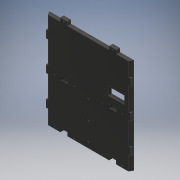
# Autodesk Inventor part: BA04
Saved by Autodesk Inventor 2017 (Build 210142000, 142)
## iProperties
Created: 2019-05-22
Part Number: BA04
Material: Wood (Cherry)
Document SubType Name: Modeling
Designer: Dell
Density: 0.63 g/cm^3
Appearance: Smooth - Black
Mass: 809.541 g
Surface Area: 2261.79 cm^2
Volume: 1284.98 cm^3
Author: Dell
Autodesk Inventor part; units mm, degrees
ref_plane "YZ Plane" through (0, 0, 0) normal (1, 0, 0) x (0, 1, 0)
ref_plane "XZ Plane" through (0, 0, 0) normal (0, 1, 0) x (-1, 0, 0)
ref_plane "XY Plane" through (0, 0, 0) normal (0, 0, 1) x (1, 0, 0)
sketch "Sketch1" plane through (0, 0, 0) normal (0, 0, 1) x (1, 0, 0)
  line L0 (0, 0) -> (303.5592, 0)
  line L1 (303.5592, 0) -> (455.3388, -262.89) construction
  line L2 (455.3388, -262.89) -> (404.5388, -350.8782)
  line L3 (404.5388, -350.8782) -> (-50.8, -87.9882) construction
  line L4 (-50.8, -87.9882) -> (0, 0) construction
  line L5 (0, 0) -> (7.3323, -12.7)
  line L6 (7.3323, -12.7) -> (296.2269, -12.7)
  line L7 (296.2269, -12.7) -> (303.5592, 0)
  dimension "d0" = 525.78
  dimension "d1" = 101.6
  dimension "d2" = 120
  dimension "d3" = 12.7
  dimension "d4" = 60
  dimension "d5" = 60
  constraints: 16 end point, 2 equal length, 2 horizontal, 2 perpendicular
  measures "d0" distance of L2.end L3.end
  measures "d1" distance of L3.end L0.start
  measures "d2" angle of L0 L4
  measures "d3" distance between parallel lines of L0 L6
  measures "d4" angle of L0 L5
  measures "d5" angle of L0 L7
extrude "Extrusion1" add sketch "Sketch1" along normal blind 342.9
sketch "Sketch2" plane through (7.3323, -12.7, 0) normal (0, -1, 0) x (1, 0, 0)
  line L0 (296.2269, 342.9) -> (-7.3323, 342.9) projected
  line L1 (43.4677, 342.9) -> (68.8677, 342.9)
  line L2 (68.8677, 342.9) -> (68.8677, 355.6)
  line L3 (68.8677, 355.6) -> (43.4677, 355.6)
  line L4 (43.4677, 355.6) -> (43.4677, 342.9)
  line L5 (220.0269, 342.9) -> (245.4269, 342.9)
  line L6 (245.4269, 342.9) -> (245.4269, 355.6)
  line L7 (245.4269, 355.6) -> (220.0269, 355.6)
  line L8 (220.0269, 355.6) -> (220.0269, 342.9)
  line L9 (-7.3323, 0) -> (-7.3323, 342.9) projected
  line L10 (296.2269, 0) -> (296.2269, 342.9) projected
  circle A0 centre (56.1677, 349.25) radius 2.25
  circle A1 centre (232.7269, 349.25) radius 2.25
  point P0 (56.1677, 355.6)
  point P1 (232.7269, 355.6)
  point P2 (68.8677, 349.25)
  point P3 (245.4269, 349.25)
  dimension "d8" = 25.4
  dimension "d9" = 12.7
  dimension "d10" = 25.4
  dimension "d11" = 12.7
  dimension "d12" = 50.8
  dimension "d13" = 50.8
  dimension "d16" = 4.5
  dimension "d17" = 4.5
  constraints: 16 end point, 4 midpoint, 4 parallel, 2 centre point, 2 horizontal, 2 horizontal alignment, 2 perpendicular, 2 point on line, 2 vertical alignment
  measures "d8" distance of L3.end L2.end
  measures "d9" distance of L2.end L1.end
  measures "d10" distance of L7.end L6.end
  measures "d11" distance of L6.end L5.end
  measures "d12" distance between parallel lines of L9 L4
  measures "d13" distance between parallel lines of L10 L6
  measures "d16" diameter of A0
  measures "d17" diameter of A1
extrude "Extrusion2" add sketch "Sketch2" against normal blind 12.7
ref_plane "Work Plane1" through (0, 0, 292.1) normal (0, 0, 1) x (1, 0, 0)
sketch "Sketch3" plane through (0, 0, 292.1) normal (0, 0, 1) x (1, 0, 0)
  line L0 (0, 0) -> (303.5592, 0) projected
  line L1 (0, 0) -> (0, -12.7)
  line L2 (296.2269, -12.7) -> (7.3323, -12.7) projected
  line L3 (0, -12.7) -> (7.3323, -12.7)
  line L4 (7.3323, -12.7) -> (0, 0) projected
  constraints: 4 end point, 1 perpendicular, 1 vertical
extrude "Extrusion3" add sketch "Sketch3" against normal blind 25.4
ref_plane "Work Plane2" through (0, 0, 50.8) normal (0, 0, -1) x (-1, 0, 0)
sketch "Sketch4" plane through (0, 0, 50.8) normal (0, 0, -1) x (-1, 0, 0)
  line L0 (0, -12.7) -> (0, 0) projected
  line L1 (-7.3323, -12.7) -> (0, 0) projected
  line L2 (-7.3323, -12.7) -> (0, -12.7) projected
extrude "Extrusion4" add sketch "Sketch4" against normal blind 25.4
ref_plane "Work Plane3" through (0, 0, 171.45) normal (0, 0, -1) x (-1, 0, 0)
sketch "Sketch5" plane through (0, 0, 171.45) normal (0, 0, -1) x (-1, 0, 0)
  line L0 (0, 0) -> (0, -12.7) projected
  line L1 (0, -12.7) -> (-7.3323, -12.7) projected
  line L2 (0, 0) -> (-7.3323, -12.7) projected
extrude "Extrusion5" add sketch "Sketch5" along normal mid plane 25.4
ref_plane "Work Plane4" through (151.7796, -12.7, 342.9) normal (-1, 0, 0) x (0, 0, 1)
mirror "Mirror1" about plane through (151.7796, -12.7, 342.9) normal (-1, 0, 0) of "Extrusion5", "Extrusion4", "Extrusion3"
sketch "Sketch6" plane through (0, 0, 0) normal (0, 0, -1) x (-1, 0, 0)
  line L0 (-76.9796, -12.7) -> (-76.9796, 0)
  line L1 (-76.9796, -6.35) -> (-64.2796, -6.35) construction
  circle A0 centre (-64.2796, -6.35) radius 2.25
  line L2 (-64.2796, -6.35) -> (-64.2796, 0) construction
  line L3 (-51.5796, -12.7) -> (-76.9796, -12.7)
  line L4 (-76.9796, 0) -> (-51.5796, 0)
  line L5 (-51.5796, 0) -> (-51.5796, -12.7)
  line L6 (-226.5796, 0) -> (-226.5796, -12.7)
  line L7 (-239.2796, 0) -> (-64.2796, 0) construction
  line L8 (-251.9796, 0) -> (-226.5796, 0)
  line L9 (-251.9796, -12.7) -> (-251.9796, 0)
  circle A1 centre (-239.2796, -6.35) radius 2.25
  line L10 (-239.2796, -6.35) -> (-239.2796, 0) construction
  line L11 (-239.2796, -6.35) -> (-226.5796, -6.35) construction
  line L12 (-226.5796, -12.7) -> (-251.9796, -12.7)
  line L13 (0, 0) -> (-303.5592, 0)
  line L14 (0, 0) -> (-303.5592, 0) projected
  point P0 (-151.7796, 0)
  dimension "d26" = 25.4
  dimension "d27" = 12.7
  dimension "d28" = 12.7
  dimension "d29" = 25.4
  dimension "d30" = 175
  dimension "d31" = 4.5
  dimension "d32" = 4.5
  constraints: 28 end point, 7 midpoint, 6 perpendicular, 4 parallel, 4 point on line, 2 centre point
  measures "d26" distance of L0.end L5.start
  measures "d27" distance of L5.start L3.start
  measures "d28" distance of L9.start L8.start
  measures "d29" distance of L8.start L6.start
  measures "d30" distance of L7.start L2.end
  measures "d31" diameter of A1
  measures "d32" diameter of A0
extrude "Extrusion6" cut sketch "Sketch6" against normal blind 12.7 contours L0 L4 L5 L3 | A0 | L6 L12 L9 L8 | A1
sketch "Sketch7" plane through (227.3592, -12.7, 355.6) normal (0, -1, 0) x (1, 0, 0)
  line L0 (-175.7796, -181.45) -> (-150.3796, -181.45)
  line L1 (-150.3796, -181.45) -> (-150.3796, -194.15)
  line L2 (-150.3796, -194.15) -> (-175.7796, -194.15)
  line L3 (-175.7796, -194.15) -> (-175.7796, -181.45)
  line L4 (-0.7796, -181.45) -> (24.6204, -181.45)
  line L5 (24.6204, -181.45) -> (24.6204, -194.15)
  line L6 (24.6204, -194.15) -> (-0.7796, -194.15)
  line L7 (-0.7796, -194.15) -> (-0.7796, -181.45)
  line L8 (-175.7796, -342.9) -> (-150.3796, -342.9) projected
  line L9 (-0.7796, -342.9) -> (24.6204, -342.9) projected
  line L10 (-227.3592, -171.45) -> (-220.0269, -171.45) projected
  point P0 (-227.3592, -355.6)
  point P1 (-163.0796, -194.15)
  point P2 (-163.0796, -342.9)
  point P3 (11.9204, -194.15)
  point P4 (11.9204, -342.9)
  dimension "d36" = 25.4
  dimension "d37" = 12.7
  dimension "d38" = 25.4
  dimension "d39" = 12.7
  dimension "d40" = 10
  constraints: 16 end point, 4 midpoint, 4 parallel, 2 horizontal, 2 perpendicular, 2 vertical alignment, 1 horizontal alignment
  measures "d36" distance of L1.end L2.end
  measures "d37" distance of L0.end L1.end
  measures "d38" distance of L5.end L6.end
  measures "d39" distance of L4.end L5.end
  measures "d40" distance between parallel lines of L10 L0
extrude "Extrusion7" cut sketch "Sketch7" against normal through all
sketch "Sketch8" plane through (227.3592, -12.7, 355.6) normal (0, -1, 0) x (1, 0, 0)
  line L0 (-150.3796, -355.6) -> (-0.7796, -355.6) construction
  line L1 (-100.9796, -355.6) -> (-50.1796, -355.6) construction
  line L2 (-50.1796, -355.6) -> (-50.1796, -181.45) construction
  line L3 (-50.1796, -181.45) -> (-100.9796, -181.45) construction
  line L4 (-100.9796, -181.45) -> (-100.9796, -355.6) construction
  circle A0 centre (-75.5796, -268.525) radius 4
  circle A1 centre (-75.5796, -201.45) radius 4
  circle A2 centre (-75.5796, -335.6) radius 4
  line L5 (-0.7796, -355.6) -> (-150.3796, -355.6)
  line L6 (-0.7796, -355.6) -> (-150.3796, -355.6) projected
  circle A3 centre (-126.3796, -187.8) radius 2.25
  circle A4 centre (-126.3796, -349.25) radius 2.25
  circle A5 centre (-24.7796, -349.25) radius 2.25
  circle A6 centre (-24.7796, -187.8) radius 2.25
  line L7 (-150.3796, -181.45) -> (-150.3796, -194.15) projected
  line L8 (-150.3796, -342.9) -> (-150.3796, -355.6) projected
  point P0 (-75.5796, -355.6)
  point P1 (-75.5796, -355.6)
  point P2 (-75.5796, -355.6)
  point P3 (-100.9796, -268.525)
  point P4 (-150.3796, -187.8)
  point P5 (-150.3796, -349.25)
  dimension "d44" = 8
  dimension "d45" = 8
  dimension "d46" = 8
  dimension "d47" = 20
  dimension "d48" = 20
  dimension "d49" = 50.8
  dimension "d59" = 4.5
  dimension "d60" = 4.5
  dimension "d61" = 4.5
  dimension "d62" = 4.5
  dimension "d63" = 25.4
  dimension "d64" = 25.4
  constraints: 12 end point, 7 centre point, 7 midpoint, 6 horizontal alignment, 5 vertical alignment, 2 coincident, 2 parallel, 1 horizontal, 1 perpendicular, 1 point on line
  measures "d44" diameter of A0
  measures "d45" diameter of A1
  measures "d46" diameter of A2
  measures "d47" distance from line of L3 A1.centre
  measures "d48" distance from line of L0 A2.centre
  measures "d49" distance of L2.end L3.end
  measures "d59" diameter of A3
  measures "d60" diameter of A4
  measures "d61" diameter of A5
  measures "d62" diameter of A6
  measures "d63" distance from line of A3.centre L4
  measures "d64" distance from line of A6.centre L2
extrude "Extrusion8" cut sketch "Sketch8" against normal through all
sketch "Sketch9" plane through (227.3592, -12.7, 355.6) normal (0, -1, 0) x (1, 0, 0)
  circle A0 centre (-197.9032, -187.8) radius 2.25
  circle A1 centre (46.744, -187.8) radius 2.25
  circle A2 centre (-197.9032, -349.25) radius 2.25
  circle A3 centre (46.744, -349.25) radius 2.25
  line L0 (-175.7796, -194.15) -> (-175.7796, -181.45) projected
  line L1 (-175.7796, -355.6) -> (-175.7796, -342.9) projected
  line L2 (24.6204, -342.9) -> (24.6204, -355.6) projected
  line L3 (-175.7796, -355.6) -> (-220.0269, -355.6) projected
  line L4 (68.8677, -355.6) -> (24.6204, -355.6) projected
  line L5 (24.6204, -181.45) -> (24.6204, -194.15) projected
  point P0 (-227.3592, -355.6)
  point P1 (-175.7796, -187.8)
  point P2 (-175.7796, -349.25)
  point P3 (24.6204, -349.25)
  point P4 (-197.9032, -355.6)
  point P5 (46.744, -355.6)
  point P6 (24.6204, -187.8)
  dimension "d52" = 4.5
  dimension "d54" = 4.5
  dimension "d55" = 4.5
  dimension "d56" = 4.5
  constraints: 6 midpoint, 4 centre point, 4 horizontal alignment, 4 vertical alignment
  measures "d52" diameter of A0
  measures "d54" diameter of A1
  measures "d55" diameter of A2
  measures "d56" diameter of A3
extrude "Extrusion9" cut sketch "Sketch9" against normal through all
sketch "Sketch11" plane through (227.3592, -12.7, 355.6) normal (0, -1, 0) x (1, 0, 0)
  line L0 (-85.5796, -112.7) -> (-65.5796, -112.7)
  line L1 (-65.5796, -112.7) -> (-65.5796, -122.7)
  line L2 (-65.5796, -122.7) -> (-85.5796, -122.7)
  line L3 (-85.5796, -122.7) -> (-85.5796, -112.7)
  line L4 (-151.1592, -12.7) -> (0, -12.7) projected
  point P0 (-227.3592, -355.6)
  point P1 (-75.5796, -112.7)
  point P2 (-75.5796, -12.7)
  dimension "d65" = 20
  dimension "d66" = 10
  dimension "d67" = 100
  constraints: 8 end point, 2 midpoint, 2 parallel, 1 horizontal, 1 perpendicular, 1 vertical alignment
  measures "d65" distance of L1.end L2.end
  measures "d66" distance of L0.end L1.end
  measures "d67" distance between parallel lines of L4 L0
extrude "Extrusion10" [suppressed]
sketch "Sketch12" plane through (76.2, 0, 342.9) normal (0, 1, 0) x (1, 0, 0)
  line L0 (206.2304, 143.75) -> (176.2304, 143.75)
  line L1 (176.2304, 143.75) -> (176.2304, 128.75)
  line L2 (176.2304, 128.75) -> (206.2304, 128.75)
  line L3 (206.2304, 128.75) -> (206.2304, 143.75)
  line L4 (0.7796, 168.75) -> (-24.6204, 168.75) projected
  line L5 (220.0269, 50.8) -> (220.0269, 0) projected
  point P0 (-76.2, 342.9)
  dimension "d70" = 30
  dimension "d71" = 15
  dimension "d72" = 25
  dimension "d76" = 13.7965
  constraints: 8 end point, 2 parallel, 1 horizontal, 1 perpendicular
  measures "d70" distance of L2.end L1.end
  measures "d71" distance of L1.end L0.end
  measures "d72" distance between parallel lines of L4 L0
  measures "d76" distance between parallel lines of L5 L3
extrude "Extrusion11" cut sketch "Sketch12" against normal through all
sketch "Sketch13" plane through (227.3592, -12.7, 355.6) normal (0, -1, 0) x (1, 0, 0)
  line L0 (25.0712, -156.45) -> (55.0712, -156.45) projected
  line L1 (55.0712, -156.45) -> (-4.9288, -156.45)
  line L2 (-4.9288, -156.45) -> (-4.9288, -126.45)
  line L3 (-4.9288, -126.45) -> (55.0712, -126.45)
  line L4 (55.0712, -126.45) -> (55.0712, -156.45)
  point P0 (-227.3592, -355.6)
  dimension "d77" = 30
  dimension "d78" = 60
  constraints: 8 end point, 2 parallel, 1 horizontal, 1 perpendicular
  measures "d77" distance of L3.end L0.end
  measures "d78" distance of L0.end L1.end
extrude "Extrusion12" cut sketch "Sketch13" against normal through all
equation "\"d27\" = d33"
equation "\"d28\" = d33"
equation "\"d33\" = 12.7"
body "Solid1"
